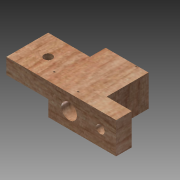
# Autodesk Inventor part: X_Top_PullySide_V2
Saved by Autodesk Inventor 2014 (Build 180170000, 170)
## iProperties
Created: 2013-12-13
Part Number: X_Top_PullySide_V2
Material: Birch
Document SubType Name: Modeling
Designer: Bram
Density: 0.512 g/cm^3
Appearance: Birch - Natural Medium Gloss
Author: Bram
Autodesk Inventor part; units mm, degrees
ref_plane "YZ Plane" through (0, 0, 0) normal (1, 0, 0) x (0, 1, 0)
ref_plane "XZ Plane" through (0, 0, 0) normal (0, 1, 0) x (-1, 0, 0)
ref_plane "XY Plane" through (0, 0, 0) normal (0, 0, 1) x (1, 0, 0)
sketch "Sketch1" plane through (0, 0, 0) normal (0, 1, 0) x (-1, 0, 0)
  line L0 (0, 0) -> (105, 0)
  line L1 (105, 0) -> (105, 30)
  line L2 (105, 30) -> (0, 30)
  line L3 (0, 30) -> (0, 0)
  line L4 (105, 0) -> (65, 0)
  line L5 (65, 0) -> (65, 15)
  line L6 (65, 15) -> (105, 15)
  line L7 (105, 15) -> (105, 0)
  line L8 (0, 15) -> (15, 15)
  line L9 (15, 15) -> (45, 15)
  circle A0 centre (15, 15) radius 4
  circle A1 centre (45, 15) radius 7.5
  dimension "d0" = 105
  dimension "d1" = 30
  dimension "d2" = 40
  dimension "d3" = 15
  dimension "d4" = 15
  dimension "d5" = 30
  dimension "d6" = 8
  dimension "d7" = 15
  constraints: 20 end point, 4 parallel, 3 perpendicular, 2 centre point, 2 coincident, 2 horizontal, 1 collinear, 1 midpoint
  measures "d0" distance of L2.end L1.end
  measures "d1" distance of L1.end L0.end
  measures "d2" distance of L5.end L6.end
  measures "d3" distance of L4.end L5.end
  measures "d4" distance of L8.start L8.end
  measures "d5" distance of L8.end L9.end
  measures "d6" diameter of A0
  measures "d7" diameter of A1
extrude "Extrusion1" add sketch "Sketch1" along normal blind 55 contours L3 L2 L1 L6 L5 L0
sketch "Sketch2" plane through (-105, 0, 30) normal (0, 0, 1) x (1, 0, 0)
  line L0 (105, 55) -> (81, 55)
  line L1 (81, 55) -> (81, 15)
  line L2 (81, 15) -> (105, 15)
  line L3 (105, 15) -> (105, 55)
  dimension "d10" = 24
  dimension "d11" = 40
  constraints: 8 end point, 2 parallel, 1 horizontal, 1 perpendicular
  measures "d10" distance of L2.end L1.end
  measures "d11" distance of L1.end L0.end
extrude "Extrusion2" cut sketch "Sketch2" against normal blind 55
sketch "Sketch3" plane through (-65, 0, 15) normal (0, 0, -1) x (-1, 0, 0)
  line L0 (40, 55) -> (0, 55)
  line L1 (0, 55) -> (0, 40)
  line L2 (0, 40) -> (40, 40)
  line L3 (40, 40) -> (40, 55)
  circle A0 centre (20, 20) radius 4
  point P0 (-65, 0)
  dimension "d15" = 15
  dimension "d16" = 8
  constraints: 8 end point, 2 parallel, 1 centre point, 1 horizontal, 1 perpendicular
  measures "d15" distance of L1.end L0.end
  measures "d16" diameter of A0
extrude "Extrusion3" cut sketch "Sketch3" against normal blind 55
body "Solid1"
